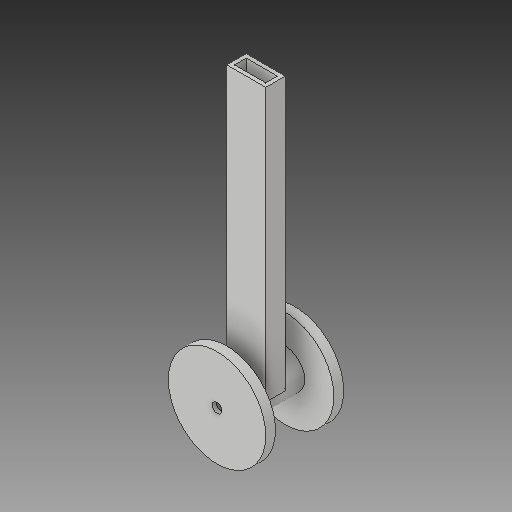
# Autodesk Inventor part: arm_proximal
Saved by Autodesk Inventor 2019 (Build 230136000, 136)
## iProperties
Created: 2019-05-02
Part Number: arm_proximal
Material: Generic
Document SubType Name: Modeling
Designer: Nathan
Density: 1 g/cm^3
Appearance: Default
Author: Nathan
Autodesk Inventor part; units mm, degrees
ref_plane "YZ Plane" through (0, 0, 0) normal (1, 0, 0) x (0, 1, 0)
ref_plane "XY Plane" through (0, 0, 0) normal (0, 0, 1) x (1, 0, 0)
sketch "Sketch1" plane through (0, 0, 0) normal (0, 0, 1) x (1, 0, 0)
  circle A0 centre (0, 0) radius 31.75
  dimension "d0" = 63.5
  constraints: 1 centre point, 1 coincident
  measures "d0" diameter of A0
extrude "Extrusion1" add sketch "Sketch1" along normal blind 6.35
sketch "Sketch2" plane through (0, 0, 6.35) normal (0, 0, 1) x (1, 0, 0)
  circle A0 centre (0, 0) radius 12.7
  dimension "d3" = 25.4
  constraints: 1 centre point, 1 coincident
  measures "d3" diameter of A0
extrude "Extrusion2" add sketch "Sketch2" along normal blind 38.1
sketch "Sketch3" plane through (0, 0, 44.45) normal (0, 0, 1) x (1, 0, 0)
  circle A0 centre (0, 0) radius 31.75
  circle A1 centre (0, 0) radius 31.75 projected
  constraints: 1 centre point, 1 coincident, 1 concentric
extrude "Extrusion3" add sketch "Sketch3" along normal blind 6.35
ref_plane "Work Plane1" through (0, 0, 0) normal (0, 1, 0) x (-1, 0, 0)
sketch "Sketch4" plane through (0, 0, 0) normal (0, 1, 0) x (-1, 0, 0)
  line L0 (-12.7, 19.05) -> (12.7, 19.05)
  line L1 (12.7, 19.05) -> (12.7, 31.75)
  line L2 (12.7, 31.75) -> (-12.7, 31.75)
  line L3 (-12.7, 31.75) -> (-12.7, 19.05)
  line L4 (-12.7, 6.35) -> (-12.7, 44.45) construction
  line L5 (12.7, 6.35) -> (12.7, 44.45) construction
  line L6 (-31.75, 44.45) -> (31.75, 44.45) construction
  line L7 (31.75, 6.35) -> (-31.75, 6.35) construction
  point P0 (0, 0)
  dimension "d9" = 25.4
  dimension "d10" = 25.4
  dimension "d11" = 12.7
  dimension "d12" = 12.7
  dimension "d13" = 12.7
  constraints: 8 end point, 2 parallel, 1 horizontal, 1 perpendicular, 1 point on line
  measures "d9" distance of L0.start L0.end
  measures "d10" distance between parallel lines of L5 L4
  measures "d11" distance between parallel lines of L6 L2
  measures "d12" distance between parallel lines of L7 L0
  measures "d13" distance between parallel lines of L2 L0
extrude "Extrusion4" add sketch "Sketch4" along normal blind 177.8
shell "Shell1" thickness 2.54 removed faces 1 at (-4.2333, 177.8, 27.5167)
sketch "Sketch5" plane through (0, 0, 50.8) normal (0, 0, 1) x (1, 0, 0)
  circle A0 centre (0, 0) radius 3.175
  dimension "d17" = 6.35
  constraints: 1 centre point, 1 coincident
  measures "d17" diameter of A0
extrude "Extrusion5" cut sketch "Sketch5" against normal through all
equation "\"d0\" = arm_proximal_gear_diameter"
equation "\"d1\" = arm_proximal_gear_thickness"
equation "\"d4\" = -2 * shoulder_wall_thickness + shoulder_width - 2 * arm_proximal_gear_thickness"
equation "\"d6\" = arm_proximal_gear_thickness"
equation "\"d9\" = d10"
equation "\"d12\" = d11"
equation "\"d13\" = arm_proximal_width"
equation "\"d14\" = arm_proximal_length"
equation "\"turntable_diameter\" = 101.6"
equation "\"turntable_thickness\" = 9.525"
equation "\"spine_diameter\" = 38.1"
equation "\"shoulder_height_offset\" = 25.4"
equation "\"shoulder_width\" = 63.5"
equation "\"shoulder_length\" = 63.5"
equation "\"shoulder_wall_thickness\" = 6.35"
equation "\"arm_proximal_gear_diameter\" = 63.5"
equation "\"shoulder_motor_gear_diameter\" = 31.75"
equation "\"arm_proximal_gear_thickness\" = 6.35"
equation "\"arm_proximal_length\" = 177.8"
equation "\"arm_proximal_width\" = 12.7"
equation "\"turntable_spur_thickness\" = 6.35"
equation "\"base_length\" = 127"
equation "\"base_width\" = 165.1"
equation "\"base_height\" = 12.7"
equation "\"retention_poles_diameter\" = 3.175"
body "Solid1"
